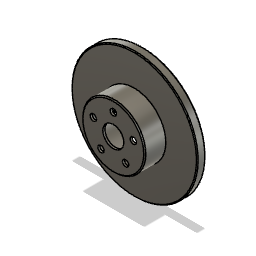
BrakeDiskProj v3 (Autodesk Fusion 360 design; units mm, degrees)
Autodesk Fusion 360 part; units mm, degrees
sketch "Sketch1" plane through (0, 0, 0) normal (0, 0, 1) x (1, 0, 0) in component "Disk"
  circle A0 centre (0, 0) radius 150
  dimension "d1" = 300
  constraint coincident A0.centre origin
  measures "d1" diameter of A0
extrude "Extrude1" add sketch "Sketch1" along normal blind 20 in component "Disk"
sketch "Sketch2" plane through (0, 0, 20) normal (0, 0, 1) x (1, 0, 0) in component "Disk"
  circle A0 centre (0, 0) radius 150
  circle A1 centre (0, 0) radius 75
  dimension "d4" = 150
  constraint coincident A0.centre A1.centre
  measures "d4" diameter of A1
extrude "Extrude2" add sketch "Sketch2" along normal blind 50 contours A1 in component "Disk"
sketch "Sketch3" plane through (0, 0, 0) normal (0, 0, -1) x (-1, 0, 0) in component "Disk"
  circle A0 centre (0, 0) radius 150
  circle A1 centre (0, 0) radius 75
  circle A2 centre (0, 0) radius 70
  dimension "d7" = -5
extrude "Extrude3" cut sketch "Sketch3" against normal up to surface (65 mm away) contours A2 in component "Disk"
chamfer "Chamfer1" distance 2.5 angle 45 1 edges at (-69.9246, -27.1212, 70) in component "Disk"
chamfer "Chamfer2" distance 2 angle 45 2 edges at (-139.8491, -54.2423, 20) (-139.8491, -54.2423, 0) in component "Disk"
sketch "Sketch4" plane through (0, 0, 70) normal (0, 0, 1) x (1, 0, 0) in component "Disk"
  circle A0 centre (0, 0) radius 72.5
  circle A1 centre (0, 0) radius 25
  dimension "d12" = 50
  constraint coincident A0.centre A1.centre
  measures "d12" diameter of A1
extrude "Extrude4" cut sketch "Sketch4" against normal up to surface (5 mm away) contours A1 in component "Disk"
sketch "Sketch5" plane through (0, 0, 70) normal (0, 0, 1) x (1, 0, 0) in component "Disk"
  circle A0 centre (0, 0) radius 25
  circle A1 centre (0, 0) radius 72.5
  point P0 (0, 50)
  dimension "d15" = 50
  measures "d15" distance of A0.centre P0
hole "Hole1" at (0, 50, 70) direction (0, 0, -1) diameter 15 depth 5 tip angle 118 in component "Disk"
pattern_circular "C-Pattern1" count 5 over 360 about axis through (0, 0, 70) along (0, 0, -1) of "Hole1" in component "Disk"
component "Disk" placed x (1, 0, 0) y (0, 1, 0) z (0, 0, 1) at (0, 0, 0)
